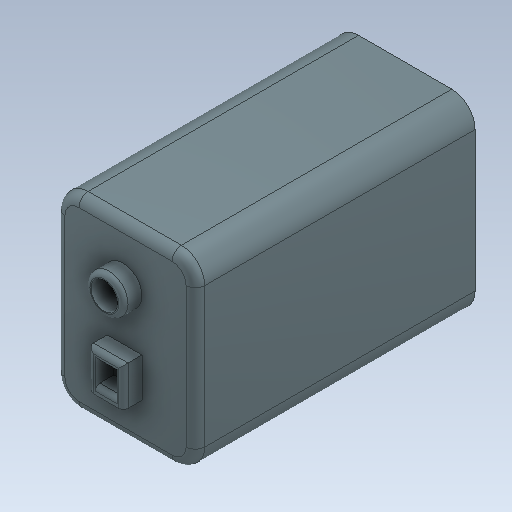
# Autodesk Inventor part: Battery1
Saved by Autodesk Inventor 2020 (Build 240168000, 168)
## iProperties
Created: 2021-06-20
Part Number: Battery1
Material: Lead
Document SubType Name: Modeling
Designer: pc
Density: 11.34 g/cm^3
Appearance: Lead
Author: pc
Autodesk Inventor part; units mm, degrees
ref_plane "YZ Plane" through (0, 0, 0) normal (1, 0, 0) x (0, 1, 0)
ref_plane "XZ Plane" through (0, 0, 0) normal (0, 1, 0) x (-1, 0, 0)
ref_plane "XY Plane" through (0, 0, 0) normal (0, 0, 1) x (1, 0, 0)
sketch "Sketch1" plane through (0, 0, 0) normal (1, 0, 0) x (0, 1, 0)
  line L0 (43.6864, 61.8662) -> (-7.1136, 61.8662)
  line L1 (-7.1136, 61.8662) -> (-7.1136, -14.3338)
  line L2 (-7.1136, -14.3338) -> (43.6864, -14.3338)
  line L3 (43.6864, -14.3338) -> (43.6864, 61.8662)
  point P0 (0, 0)
  constraints: 8 end point, 2 parallel, 1 horizontal, 1 perpendicular
extrude "Extrusion1" add sketch "Sketch1" along normal blind 38.1
fillet "Fillet1" radius 6.35 4 edges at (38.1, 43.6864, 23.7662) (0, 43.6864, 23.7662) (38.1, -7.1136, 23.7662) (0, -7.1136, 23.7662)
sketch "Sketch2" plane through (0, -0.7636, 61.8662) normal (0, 0, 1) x (1, 0, 0)
  circle A0 centre (18.3636, 29.6461) radius 5.1979
  line L0 (14.0847, 15.7397) -> (23.5615, 15.7397)
  line L1 (23.5615, 15.7397) -> (23.5615, 5.0424)
  line L2 (23.5615, 5.0424) -> (14.0847, 5.0424)
  line L3 (14.0847, 5.0424) -> (14.0847, 15.7397)
  point P0 (0, 0.7636)
  constraints: 8 end point, 2 parallel, 1 centre point, 1 horizontal, 1 perpendicular
extrude "Extrusion2" add sketch "Sketch2" along normal blind 5.08
sketch "Sketch3" plane through (18.3636, 28.8825, 66.9462) normal (0, 0, 1) x (1, 0, 0)
  circle A0 centre (0, 0) radius 3.6755
  point P0 (-18.3636, -28.8825)
  constraints: 1 centre point
extrude "Extrusion3" cut sketch "Sketch3" against normal blind 5.08
sketch "Sketch4" plane through (0, -0.7636, 66.9462) normal (0, 0, 1) x (1, 0, 0)
  line L0 (15.8676, 13.9568) -> (21.9293, 13.9568)
  line L1 (21.9293, 13.9568) -> (21.9293, 7.1819)
  line L2 (21.9293, 7.1819) -> (15.8676, 7.1819)
  line L3 (15.8676, 7.1819) -> (15.8676, 13.9568)
  point P0 (0, 0.7636)
  constraints: 8 end point, 2 parallel, 1 horizontal, 1 perpendicular
extrude "Extrusion4" cut sketch "Sketch4" against normal blind 5.08
fillet "Fillet2" radius 1.27 4 edges at (18.8231, 14.9761, 66.9462) (23.5615, 9.6275, 66.9462) (18.8984, 6.4183, 66.9462) (14.0847, 9.6275, 66.9462)
fillet "Fillet3" radius 1.27 1 edges at (13.1657, 28.8825, 66.9462)
fillet "Fillet4" radius 2.54 8 edges at (36.2401, 41.8266, 61.8662) (38.1, 18.2864, 61.8662) (36.2401, -5.2537, 61.8662) (19.05, -7.1136, 61.8662) (1.8599, -5.2537, 61.8662) (0, 18.2864, 61.8662) (1.8599, 41.8266, 61.8662) (19.05, 43.6864, 61.8662)
body "Solid1"
